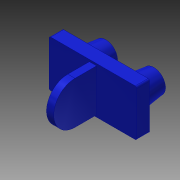
# Autodesk Inventor part: HIPS
Saved by Autodesk Inventor 2015 (Build 190159000, 159)
## iProperties
Created: 2012-05-01
Part Number: HIPS
Material: 250
Document SubType Name: Modeling
Mass: 3.28465 g
Surface Area: 5.22387 cm^2
Volume: 0.418427 cm^3
Density: 7.85 g/cm^3
Appearance: Steel
Autodesk Inventor part; units mm, degrees
ref_plane "YZ Plane" through (0, 0, 0) normal (1, 0, 0) x (0, 1, 0)
ref_plane "XZ Plane" through (0, 0, 0) normal (0, 1, 0) x (-1, 0, 0)
ref_plane "XY Plane" through (0, 0, 0) normal (0, 0, 1) x (1, 0, 0)
sketch "Sketch1" plane through (0, 0, 0) normal (0, 0, 1) x (1, 0, 0)
  line L0 (-7.3, 3.875) -> (7.3, 3.875)
  line L1 (7.3, 3.875) -> (7.3, -3.875)
  line L2 (7.3, -3.875) -> (-7.3, -3.875)
  line L3 (-7.3, -3.875) -> (-7.3, 3.875)
  point P0 (0, 0)
  point P1 (-7.3, 0)
  point P2 (0, 3.875)
  dimension "d0" = 14.6
  dimension "d1" = 7.75
  constraints: 8 end point, 2 midpoint, 2 parallel, 1 horizontal, 1 horizontal alignment, 1 perpendicular, 1 vertical alignment
  measures "d0" distance of L0.start L0.end
  measures "d1" distance of L2.end L0.start
extrude "Extrusion1" add sketch "Sketch1" along normal mid plane 2.15
fillet "Fillet1" radius 0.25 4 edges at (-7.3, 3.875, 0) (-7.3, -3.875, 0) (7.3, 3.875, 0) (7.3, -3.875, 0)
sketch "Sketch2" plane through (0, 0, 0) normal (1, 0, 0) x (0, 1, 0)
  line L0 (3.625, 1.075) -> (-3.625, 1.075) construction
  line L1 (3.54, 1.075) -> (3.54, 4.675)
  arc A0 (3.54, 4.675) -> (-3.54, 4.675) centre (0, 4.675) ccw
  line L2 (-3.54, 4.675) -> (-3.54, 1.075)
  line L3 (-3.54, 1.075) -> (3.54, 1.075)
  point P0 (0, 0)
  dimension "d5" = 3.6
  dimension "d6" = 7.08
  constraints: 6 end point, 2 perpendicular, 2 point on circle, 2 point on line, 2 tangent, 1 centre point, 1 collinear, 1 vertical alignment
  measures "d5" distance of L2.start L2.end
  measures "d6" distance between parallel lines of L1 L2
extrude "Extrusion2" add sketch "Sketch2" along normal mid plane 1.2
sketch "Sketch3" plane through (0, 0, 0) normal (0, 1, 0) x (-1, 0, 0)
  line L0 (7.05, -1.075) -> (-7.05, -1.075) construction
  line L1 (-4, -1.075) -> (-6.44, -1.075)
  line L2 (-6.44, -1.075) -> (-5.94, -5.075)
  line L3 (-5.94, -5.075) -> (-4, -5.075)
  line L4 (-4, -5.075) -> (-4, -1.075)
  point P0 (0, 0)
  dimension "d9" = 4.88
  dimension "d10" = 3.88
  dimension "d11" = 4
  dimension "d12" = 4
  constraints: 8 end point, 2 point on line, 1 parallel, 1 perpendicular
  measures "d9" diameter of L1.end L4
  measures "d10" diameter of L2.end L4
  measures "d11" distance between parallel lines of L0 L3
  measures "d12" horizontal distance of point (0, 0) L1.start
revolve "Revolution1" add sketch "Sketch3" angle 360 about axis through (4, 0, -5.075) along (0, 0, 1)
mirror "Mirror1" about plane through (0, 0, 0) normal (1, 0, 0) of "Revolution1"
body "Solid1"
